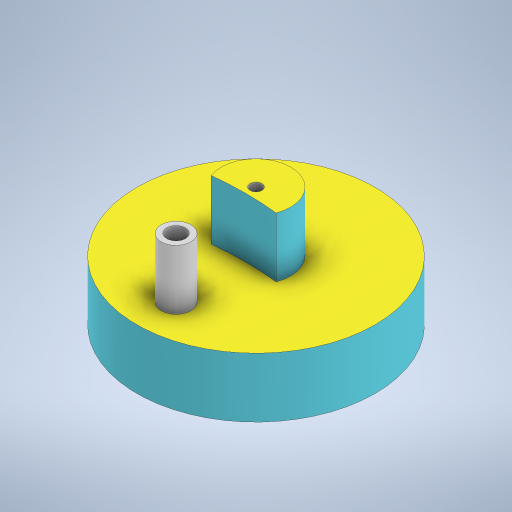
# Autodesk Inventor part: Geneva Circle arc 12
Saved by Autodesk Inventor 2023 (Build 270158000, 158)
## iProperties
Created: 2022-10-22
Part Number: Geneva Circle arc 12
Material: Generic
Document SubType Name: Modeling
Designer: annah
Density: 1 g/cm^3
Appearance: Default
Author: annah
Autodesk Inventor part; units mm, degrees
ref_plane "YZ Plane" through (0, 0, 0) normal (1, 0, 0) x (0, 1, 0)
ref_plane "XZ Plane" through (0, 0, 0) normal (0, 1, 0) x (-1, 0, 0)
ref_plane "XY Plane" through (0, 0, 0) normal (0, 0, 1) x (1, 0, 0)
sketch "Sketch1" plane through (0, 0, 0) normal (0, 1, 0) x (-1, 0, 0)
  circle A0 centre (0, 0) radius 100
  line L0 (0, 0) -> (18.5658, -69.2885)
  line L1 (0, 0) -> (0, -103.5276)
  arc A1 (24.6448, -72.6673) -> (14.9907, -75.2542) centre (0, 0) ccw
  circle A2 centre (25.8819, -96.5926) radius 5
  arc A3 (24.729, -72.9816) -> (15.0747, -75.5678) centre (19.8599, -74.1181) ccw
  line L2 (30.6777, -95.1782) -> (24.6448, -72.6673)
  line L3 (21.0523, -97.8867) -> (14.9907, -75.2542)
  circle A4 centre (0, -103.5276) radius 11.6229
  line L4 (21.0523, -97.8867) -> (25.8819, -96.5926)
  arc A5 (-25.8819, -96.5926) -> (26.7197, -101.5219) centre (0, -103.5276) ccw
  circle A6 centre (0, -103.5276) radius 39.9
  arc A7 (57.9067, -50.8394) -> (50.8389, -57.9063) centre (54.2582, -54.2582) ccw
  line L5 (67.1751, -74.2462) -> (50.6094, -57.6767)
  line L6 (74.1567, -67.0879) -> (57.6767, -50.6094)
  circle A8 centre (70.7107, -70.7107) radius 5
  circle A9 centre (51.7638, -89.6575) radius 11.6229
  arc A10 (75.5684, -15.0748) -> (72.9809, -24.7289) centre (74.1181, -19.8599) ccw
  line L7 (95.2985, -30.7115) -> (72.6673, -24.6448)
  line L8 (97.7655, -21.0214) -> (75.2542, -14.9907)
  circle A11 centre (96.5926, -25.8819) radius 5
  circle A12 centre (89.6575, -51.7638) radius 11.6229
  arc A13 (72.9816, 24.729) -> (75.5678, 15.0747) centre (74.1181, 19.8599) ccw
  line L9 (97.8867, 21.0523) -> (75.2542, 14.9907)
  line L10 (95.1782, 30.6777) -> (72.6673, 24.6448)
  circle A14 centre (96.5926, 25.8819) radius 5
  circle A15 centre (103.5276, 0) radius 11.6229
  arc A16 (50.8394, 57.9067) -> (57.9063, 50.8389) centre (54.2582, 54.2582) ccw
  line L11 (74.2462, 67.1751) -> (57.6767, 50.6094)
  line L12 (67.0879, 74.1567) -> (50.6094, 57.6767)
  circle A17 centre (70.7107, 70.7107) radius 5
  circle A18 centre (89.6575, 51.7638) radius 11.6229
  arc A19 (15.0748, 75.5684) -> (24.7289, 72.9809) centre (19.8599, 74.1181) ccw
  line L13 (30.7115, 95.2985) -> (24.6448, 72.6673)
  line L14 (21.0214, 97.7655) -> (14.9907, 75.2542)
  circle A20 centre (25.8819, 96.5926) radius 5
  circle A21 centre (51.7638, 89.6575) radius 11.6229
  arc A22 (-24.729, 72.9816) -> (-15.0747, 75.5678) centre (-19.8599, 74.1181) ccw
  line L15 (-21.0523, 97.8867) -> (-14.9907, 75.2542)
  line L16 (-30.6777, 95.1782) -> (-24.6448, 72.6673)
  circle A23 centre (-25.8819, 96.5926) radius 5
  circle A24 centre (0, 103.5276) radius 11.6229
  arc A25 (-57.9067, 50.8394) -> (-50.8389, 57.9063) centre (-54.2582, 54.2582) ccw
  line L17 (-67.1751, 74.2462) -> (-50.6094, 57.6767)
  line L18 (-74.1567, 67.0879) -> (-57.6767, 50.6094)
  circle A26 centre (-70.7107, 70.7107) radius 5
  circle A27 centre (-51.7638, 89.6575) radius 11.6229
  arc A28 (-75.5684, 15.0748) -> (-72.9809, 24.7289) centre (-74.1181, 19.8599) ccw
  line L19 (-95.2985, 30.7115) -> (-72.6673, 24.6448)
  line L20 (-97.7655, 21.0214) -> (-75.2542, 14.9907)
  circle A29 centre (-96.5926, 25.8819) radius 5
  circle A30 centre (-89.6575, 51.7638) radius 11.6229
  arc A31 (-72.9816, -24.729) -> (-75.5678, -15.0747) centre (-74.1181, -19.8599) ccw
  line L21 (-97.8867, -21.0523) -> (-75.2542, -14.9907)
  line L22 (-95.1782, -30.6777) -> (-72.6673, -24.6448)
  circle A32 centre (-96.5926, -25.8819) radius 5
  circle A33 centre (-103.5276, 0) radius 11.6229
  arc A34 (-50.8394, -57.9067) -> (-57.9063, -50.8389) centre (-54.2582, -54.2582) ccw
  line L23 (-74.2462, -67.1751) -> (-57.6767, -50.6094)
  line L24 (-67.0879, -74.1567) -> (-50.6094, -57.6767)
  circle A35 centre (-70.7107, -70.7107) radius 5
  circle A36 centre (-89.6575, -51.7638) radius 11.6229
  arc A37 (-15.0748, -75.5684) -> (-24.7289, -72.9809) centre (-19.8599, -74.1181) ccw
  line L25 (-30.7115, -95.2985) -> (-24.6448, -72.6673)
  line L26 (-21.0214, -97.7655) -> (-14.9907, -75.2542)
  circle A38 centre (-25.8819, -96.5926) radius 5
  circle A39 centre (-51.7638, -89.6575) radius 11.6229
  circle A40 centre (0, 0) radius 5
  circle A41 centre (0, -103.5276) radius 2
  circle A42 centre (0, -76.7327) radius 5
  point P0 (50.7227, -50.7227)
  point P1 (73.9009, -74.5607)
  point P2 (69.2885, -18.5658)
  point P3 (101.2804, -27.621)
  point P4 (69.2885, 18.5658)
  point P5 (101.5219, 26.7197)
  point P6 (50.7227, 50.7227)
  point P7 (74.5607, 73.9009)
  point P8 (18.5658, 69.2885)
  point P9 (27.621, 101.2804)
  point P10 (-18.5658, 69.2885)
  point P11 (-26.7197, 101.5219)
  point P12 (-50.7227, 50.7227)
  point P13 (-73.9009, 74.5607)
  point P14 (-69.2885, 18.5658)
  point P15 (-101.2804, 27.621)
  point P16 (-69.2885, -18.5658)
  point P17 (-101.5219, -26.7197)
  point P18 (-50.7227, -50.7227)
  point P19 (-74.5607, -73.9009)
  point P20 (-18.5658, -69.2885)
  point P21 (-27.621, -101.2804)
  point P22 (40.2917, -91.5236)
  point P23 (59.1159, -80.6555)
  point P24 (67.0867, -74.1578)
  point P25 (80.6555, -59.1159)
  point P26 (91.5236, -40.2917)
  point P27 (95.1777, -30.6791)
  point P28 (99.4077, -10.8682)
  point P29 (99.4077, 10.8682)
  point P30 (97.7659, 21.0199)
  point P31 (91.5236, 40.2917)
  point P32 (80.6555, 59.1159)
  point P33 (74.1578, 67.0867)
  point P34 (59.1159, 80.6555)
  point P35 (40.2917, 91.5236)
  point P36 (30.6791, 95.1777)
  point P37 (10.8682, 99.4077)
  point P38 (-10.8682, 99.4077)
  point P39 (-21.0199, 97.7659)
  point P40 (-40.2917, 91.5236)
  point P41 (-59.1159, 80.6555)
  point P42 (-67.0867, 74.1578)
  point P43 (-80.6555, 59.1159)
  point P44 (-91.5236, 40.2917)
  point P45 (-95.1777, 30.6791)
  point P46 (-99.4077, 10.8682)
  point P47 (-99.4077, -10.8682)
  point P48 (-97.7659, -21.0199)
  point P49 (-91.5236, -40.2917)
  point P50 (-80.6555, -59.1159)
  point P51 (-74.1578, -67.0867)
  point P52 (-59.1159, -80.6555)
  point P53 (-40.2917, -91.5236)
  point P54 (-30.6791, -95.1777)
  point P55 (-10.8682, -99.4077)
  point P56 (10.8682, -99.4077)
  point P57 (21.0199, -97.7659)
  point P58 (-10.8682, -99.4077)
  point P59 (10.8682, -99.4077)
  dimension "d2" = 200
  dimension "d3" = 15
  dimension "d4" = 10
  dimension "d5" = 10
  dimension "d6" = 79.8
  dimension "d7" = 360
  dimension "d8" = 10
  dimension "d9" = 4
  dimension "d14" = 10
  constraints: 104 point on circle, 54 end point, 43 centre point, 26 point on line, 8 coincident, 1 vertical, 193 other
  measures "d2" diameter of A0
  measures "d3" angle of L1 L0
  measures "d4" diameter of A2
  measures "d5" diameter of A3
  measures "d6" diameter of A6
  measures "d8" diameter of A40
  measures "d9" diameter of A41
  measures "d14" diameter of A42
extrude "Extrusion1" add sketch "Sketch1" along normal blind 20 contours A0 A4
extrude "Extrusion2" add sketch "Sketch1" against normal blind 20 contours A0 A38 | A5 A38 L25 A0 | A0 A38 A5 | L26 A37 A1 A42 L1 A4 A0 | A38 L25 A37 A1 L26 | A0 A4 A2 A5 A38 | L25 A38 A5 A2 A0 A6 | A0 A6 A1 A37 L25 | A4 L1 A0 | A41 | A0 A4 | A2 L4 A0 | L1 A4 A0 | L1 A42 A1 A3 L3 A0 A4 | A37 A6 L1 A42 A1 | A1 A37 A6 | A6 A37 A1 | A2 A0 L4 | A42 A1 L1 | L1 A1 A42 | A42 L1 A1 | A0 L2 A3 A1 A6 | A2 A0 | L3 A3 A6 L2 A2 | L1 A42 A1 | L1 A6 L0 A3 A1 A42 | A1 A3 A6 | A3 L3 | A6 A3 L0
sketch "Sketch2" plane through (0, 0, -103.5276) normal (0, 1, 0) x (1, 0, 0)
  circle A0 centre (0, 0) radius 2 projected
  circle A1 centre (0, 0) radius 2.5
  point P0 (0, -103.5276)
  constraints: 1 centre point, 1 coincident
extrude "Extrusion3" cut sketch "Sketch2" against normal blind 20 contours A0
extrude "Extrusion5" add sketch "Sketch1" along normal blind 20 contours A42 A1 L1 | L1 A1 A42 | A42 L1 A1 | L1 A42 A1
sketch "Sketch4" plane through (0, 20, -76.7327) normal (0, 1, 0) x (1, 0, 0)
  circle A0 centre (0, 0) radius 3.15
  point P0 (0, -76.7327)
  dimension "d22" = 6.3
  constraints: 1 centre point
  measures "d22" diameter of A0
extrude "Extrusion6" cut sketch "Sketch4" against normal blind 20
body "Solid1"
